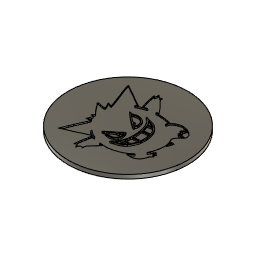
gengar v2 (Autodesk Fusion 360 design; units mm, degrees)
Autodesk Fusion 360 part; units mm, degrees
(part 1 of 2)
sketch "Sketch1" plane through (0, 0, 0) normal (0, 0, 1) x (1, 0, 0)
  circle A0 centre (0, 0) radius 44.85
  dimension "d1" = 89.7
  constraint coincident A0.centre origin
  measures "d1" diameter of A0
extrude "Extrude1" add sketch "Sketch1" along normal blind 2
sketch "Sketch2" plane through (0, 0, 2) normal (0, 0, 1) x (-1, 0, 0)
  circle A0 centre (0, 0) radius 44.85
  line L0 (0, 0) -> (35, 0) construction
  line L1 (35, 0) -> (35, 35) construction
  spline S0 degree 3 poles (24.9655, 28.3529) (24.8458, 28.3933) (24.5786, 28.3486) (24.2945, 28.2347) knots 0 0 0 0 1 1 1 1
  spline S1 degree 3 poles (24.2945, 28.2347) (24.0383, 28.1309) (22.2564, 27.4299) (20.3388, 26.6689) knots 0 0 0 0 1 1 1 1
  spline S2 degree 3 poles (20.3388, 26.6689) (18.4212, 25.908) (16.711, 25.212) (16.545, 25.1201) knots 0 0 0 0 1 1 1 1
  spline S3 degree 3 poles (16.545, 25.1201) (16.3696, 25.0248) (15.5285, 24.6241) (14.6653, 24.2259) knots 0 0 0 0 1 1 1 1
  spline S4 degree 3 poles (14.6653, 24.2259) (11.416, 22.7388) (8.4179, 21.3116) (7.8616, 20.9936) knots 0 0 0 0 1 1 1 1
  line L2 (7.8616, 20.9936) -> (7.5666, 20.8232)
  line L3 (7.5666, 20.8232) -> (7.7132, 21.2861)
  spline S5 degree 3 poles (7.7132, 21.2861) (7.9347, 21.9757) (8.1275, 22.8019) (8.1956, 23.3937) knots 0 0 0 0 1 1 1 1
  spline S6 degree 3 poles (8.1956, 23.3937) (8.2284, 23.6786) (8.3176, 24.0681) (8.3842, 24.2603) knots 0 0 0 0 1 1 1 1
  spline S7 degree 3 poles (8.3842, 24.2603) (8.4507, 24.4526) (8.5341, 24.8294) (8.5702, 25.1051) knots 0 0 0 0 1 1 1 1
  spline S8 degree 3 poles (8.5702, 25.1051) (8.6005, 25.3681) (8.6687, 25.7289) (8.7142, 25.8925) knots 0 0 0 0 1 1 1 1
  spline S9 degree 3 poles (8.7142, 25.8925) (8.8203, 26.2356) (8.9339, 26.991) (8.9994, 27.6763) knots 0 0 0 0 1 1 1 1
  spline S10 degree 3 poles (8.9994, 27.6763) (9.017, 27.9453) (9.0565, 28.3271) (9.0792, 28.5244) knots 0 0 0 0 1 1 1 1
  spline S11 degree 3 poles (9.0792, 28.5244) (9.1078, 28.7343) (9.1111, 28.956) (9.0934, 29.0336) knots 0 0 0 0 1 1 1 1
  spline S12 degree 3 poles (9.0934, 29.0336) (9.0757, 29.1111) (9.0975, 29.3396) (9.1481, 29.547) knots 0 0 0 0 1 1 1 1
  spline S13 degree 3 poles (9.1481, 29.547) (9.1927, 29.7417) (9.2609, 30.1026) (9.2886, 30.3437) knots 0 0 0 0 1 1 1 1
  spline S14 degree 3 poles (9.2886, 30.3437) (9.329, 30.5789) (9.4241, 30.981) (9.4983, 31.239) knots 0 0 0 0 1 1 1 1
  spline S15 degree 3 poles (9.4983, 31.239) (9.6549, 31.7895) (9.5873, 32.3214) (9.3368, 32.5768) knots 0 0 0 0 1 1 1 1
  spline S16 degree 3 poles (9.3368, 32.5768) (9.1024, 32.817) (8.6363, 32.7418) (7.9788, 32.3555) knots 0 0 0 0 1 1 1 1
  spline S17 degree 3 poles (7.9788, 32.3555) (7.7024, 32.1919) (7.4563, 32.0603) (7.4403, 32.0755) knots 0 0 0 0 1 1 1 1
  spline S18 degree 3 poles (7.4403, 32.0755) (7.415, 32.0873) (7.3854, 32.255) (7.3643, 32.4573) knots 0 0 0 0 1 1 1 1
  spline S19 degree 3 poles (7.3643, 32.4573) (7.3507, 32.7254) (7.2647, 32.9041) (7.0547, 33.1637) knots 0 0 0 0 1 1 1 1
  spline S20 degree 3 poles (7.0547, 33.1637) (6.9029, 33.3499) (6.7199, 33.6508) (6.6591, 33.8177) knots 0 0 0 0 1 1 1 1
  line L4 (6.6591, 33.8177) -> (6.5444, 34.133)
  line L5 (6.5444, 34.133) -> (5.7099, 33.8292)
  line L6 (5.7099, 33.8292) -> (4.8847, 33.5289)
  line L7 (4.8847, 33.5289) -> (4.7862, 33.136)
  spline S21 degree 3 poles (4.7862, 33.136) (4.6506, 32.6142) (4.2876, 31.7365) (4.1948, 31.7028) knots 0 0 0 0 1 1 1 1
  spline S22 degree 3 poles (4.1948, 31.7028) (4.1485, 31.6859) (3.807, 31.8451) (3.4268, 32.0532) knots 0 0 0 0 1 1 1 1
  spline S23 degree 3 poles (3.4268, 32.0532) (2.7295, 32.4399) (2.3973, 32.4871) (2.0855, 32.2475) knots 0 0 0 0 1 1 1 1
  spline S24 degree 3 poles (2.0855, 32.2475) (1.9203, 32.1244) (1.8757, 31.8142) (1.754, 30.1003) knots 0 0 0 0 1 1 1 1
  spline S25 degree 3 poles (1.754, 30.1003) (1.7271, 29.7126) (1.6438, 29.4512) (1.4803, 29.2657) knots 0 0 0 0 1 1 1 1
  spline S26 degree 3 poles (1.4803, 29.2657) (1.3437, 29.1215) (1.1424, 28.8382) (1.0387, 28.6325) knots 0 0 0 0 1 1 1 1
  spline S27 degree 3 poles (1.0387, 28.6325) (0.9224, 28.4327) (0.796, 28.2606) (0.7682, 28.2505) knots 0 0 0 0 1 1 1 1
  spline S28 degree 3 poles (0.7682, 28.2505) (0.7311, 28.237) (0.239, 27.7429) (-0.3442, 27.1526) knots 0 0 0 0 1 1 1 1
  spline S29 degree 3 poles (-0.3442, 27.1526) (-0.9181, 26.5657) (-1.4617, 26.0109) (-1.5468, 25.9274) knots 0 0 0 0 1 1 1 1
  spline S30 degree 3 poles (-1.5468, 25.9274) (-1.6319, 25.8439) (-1.792, 25.6491) (-1.9125, 25.4898) knots 0 0 0 0 1 1 1 1
  spline S31 degree 3 poles (-1.9125, 25.4898) (-2.0237, 25.3338) (-2.269, 25.0555) (-2.4451, 24.8759) knots 0 0 0 0 1 1 1 1
  spline S32 degree 3 poles (-2.4451, 24.8759) (-2.6179, 24.687) (-2.7586, 24.4678) (-2.7594, 24.3835) knots 0 0 0 0 1 1 1 1
  spline S33 degree 3 poles (-2.7594, 24.3835) (-2.7602, 24.2992) (-2.8234, 24.2132) (-2.8976, 24.1862) knots 0 0 0 0 1 1 1 1
  spline S34 degree 3 poles (-2.8976, 24.1862) (-2.9718, 24.1592) (-3.212, 23.9248) (-3.4235, 23.6693) knots 0 0 0 0 1 1 1 1
  spline S35 degree 3 poles (-3.4235, 23.6693) (-3.635, 23.4138) (-3.8777, 23.1575) (-3.9822, 23.0984) knots 0 0 0 0 1 1 1 1
  spline S36 degree 3 poles (-3.9822, 23.0984) (-4.0775, 23.0428) (-4.7156, 22.9785) (-5.4018, 22.9598) knots 0 0 0 0 1 1 1 1
  spline S37 degree 3 poles (-5.4018, 22.9598) (-7.9965, 22.8764) (-8.3724, 22.813) (-11.5907, 21.9042) knots 0 0 0 0 1 1 1 1
  spline S38 degree 3 poles (-11.5907, 21.9042) (-13.5606, 21.3447) (-16.0531, 20.3745) (-16.4703, 19.9917) knots 0 0 0 0 1 1 1 1
  spline S39 degree 3 poles (-16.4703, 19.9917) (-16.7964, 19.705) (-17.2542, 19.6644) (-18.0837, 19.8664) knots 0 0 0 0 1 1 1 1
  spline S40 degree 3 poles (-18.0837, 19.8664) (-19.312, 20.1544) (-19.4908, 20.1838) (-20.0969, 20.2047) knots 0 0 0 0 1 1 1 1
  spline S41 degree 3 poles (-20.0969, 20.2047) (-21.2189, 20.2583) (-22.0602, 20.0887) (-23.9517, 19.4002) knots 0 0 0 0 1 1 1 1
  line L8 (-23.9517, 19.4002) -> (-25.7133, 18.759)
  line L9 (-25.7133, 18.759) -> (-26.4592, 18.0675)
  spline S42 degree 3 poles (-26.4592, 18.0675) (-26.8671, 17.6881) (-27.4089, 17.0708) (-27.6643, 16.7049) knots 0 0 0 0 1 1 1 1
  spline S43 degree 3 poles (-27.6643, 16.7049) (-28.1269, 16.043) (-28.896, 14.377) (-28.8285, 14.1916) knots 0 0 0 0 1 1 1 1
  spline S44 degree 3 poles (-28.8285, 14.1916) (-28.8083, 14.136) (-28.8402, 13.8198) (-28.9093, 13.4902) knots 0 0 0 0 1 1 1 1
  spline S45 degree 3 poles (-28.9093, 13.4902) (-28.9968, 13.0383) (-29.1004, 12.8326) (-29.3238, 12.6673) knots 0 0 0 0 1 1 1 1
  spline S46 degree 3 poles (-29.3238, 12.6673) (-29.4797, 12.5476) (-29.7915, 12.1926) (-30.0266, 11.8865) knots 0 0 0 0 1 1 1 1
  spline S47 degree 3 poles (-30.0266, 11.8865) (-30.2491, 11.5745) (-30.4698, 11.3157) (-30.5069, 11.3022) knots 0 0 0 0 1 1 1 1
  spline S48 degree 3 poles (-30.5069, 11.3022) (-30.544, 11.2887) (-30.6923, 11.0037) (-30.8389, 10.6563) knots 0 0 0 0 1 1 1 1
  spline S49 degree 3 poles (-30.8389, 10.6563) (-31.1556, 9.911) (-31.0847, 9.6008) (-30.5764, 9.5023) knots 0 0 0 0 1 1 1 1
  line L10 (-30.5764, 9.5023) -> (-30.2122, 9.4249)
  line L11 (-30.2122, 9.4249) -> (-30.5678, 9.075)
  spline S50 degree 3 poles (-30.5678, 9.075) (-30.8535, 8.7925) (-30.9209, 8.6314) (-30.9435, 8.2032) knots 0 0 0 0 1 1 1 1
  spline S51 degree 3 poles (-30.9435, 8.2032) (-30.9989, 7.259) (-30.8488, 7.1351) (-29.8862, 7.3175) knots 0 0 0 0 1 1 1 1
  spline S52 degree 3 poles (-29.8862, 7.3175) (-29.5414, 7.38) (-29.243, 7.4256) (-29.2303, 7.4197) knots 0 0 0 0 1 1 1 1
  spline S53 degree 3 poles (-29.2303, 7.4197) (-29.205, 7.4079) (-29.2269, 7.1795) (-29.2757, 6.9097) knots 0 0 0 0 1 1 1 1
  spline S54 degree 3 poles (-29.2757, 6.9097) (-29.3153, 6.6433) (-29.3185, 6.3061) (-29.2679, 6.167) knots 0 0 0 0 1 1 1 1
  spline S55 degree 3 poles (-29.2679, 6.167) (-29.089, 5.6756) (-28.3691, 5.7171) (-27.7969, 6.2509) knots 0 0 0 0 1 1 1 1
  spline S56 degree 3 poles (-27.7969, 6.2509) (-27.4649, 6.5503) (-26.965, 6.7637) (-26.911, 6.6153) knots 0 0 0 0 1 1 1 1
  spline S57 degree 3 poles (-26.911, 6.6153) (-26.8908, 6.5597) (-26.9539, 6.3582) (-27.0424, 6.1685) knots 0 0 0 0 1 1 1 1
  spline S58 degree 3 poles (-27.0424, 6.1685) (-27.2513, 5.7039) (-27.6445, 4.1013) (-27.7968, 3.0484) knots 0 0 0 0 1 1 1 1
  spline S59 degree 3 poles (-27.7968, 3.0484) (-27.9752, 1.8074) (-27.9886, 1.6135) (-28.0356, 0.9349) knots 0 0 0 0 1 1 1 1
  spline S60 degree 3 poles (-28.0356, 0.9349) (-28.0734, 0.4906) (-28.1534, 0.22) (-28.338, 0.0058) knots 0 0 0 0 1 1 1 1
  spline S61 degree 3 poles (-28.338, 0.0058) (-28.4736, -0.1696) (-28.5815, -0.3348) (-28.568, -0.3719) knots 0 0 0 0 1 1 1 1
  spline S62 degree 3 poles (-28.568, -0.3719) (-28.5545, -0.409) (-28.632, -0.5422) (-28.7441, -0.667) knots 0 0 0 0 1 1 1 1
  spline S63 degree 3 poles (-28.7441, -0.667) (-28.8562, -0.7918) (-29.0466, -1.1341) (-29.1729, -1.4216) knots 0 0 0 0 1 1 1 1
  spline S64 degree 3 poles (-29.1729, -1.4216) (-29.3052, -1.7218) (-29.5108, -2.1956) (-29.6464, -2.4865) knots 0 0 0 0 1 1 1 1
  spline S65 degree 3 poles (-29.6464, -2.4865) (-30.3406, -4.0411) (-30.3889, -5.9278) (-29.7296, -6.1813) knots 0 0 0 0 1 1 1 1
  spline S66 degree 3 poles (-29.7296, -6.1813) (-29.6158, -6.2344) (-29.0653, -6.2755) (-28.5123, -6.2948) knots 0 0 0 0 1 1 1 1
  spline S67 degree 3 poles (-28.5123, -6.2948) (-26.6256, -6.3431) (-26.4461, -6.4037) (-26.0437, -7.1918) knots 0 0 0 0 1 1 1 1
  spline S68 degree 3 poles (-26.0437, -7.1918) (-25.8194, -7.6352) (-25.8126, -7.6537) (-26.0511, -8.066) knots 0 0 0 0 1 1 1 1
  spline S69 degree 3 poles (-26.0511, -8.066) (-26.1884, -8.2945) (-26.3754, -8.6461) (-26.4791, -8.8518) knots 0 0 0 0 1 1 1 1
  spline S70 degree 3 poles (-26.4791, -8.8518) (-26.6383, -9.1933) (-28.4257, -11.0619) (-29.2104, -11.7045) knots 0 0 0 0 1 1 1 1
  spline S71 degree 3 poles (-29.2104, -11.7045) (-30.065, -12.4145) (-30.5646, -13.3209) (-30.5585, -14.1167) knots 0 0 0 0 1 1 1 1
  spline S72 degree 3 poles (-30.5585, -14.1167) (-30.555, -14.3569) (-30.3381, -15.097) (-29.9661, -16.1481) knots 0 0 0 0 1 1 1 1
  spline S73 degree 3 poles (-29.9661, -16.1481) (-29.3814, -17.7834) (-29.3654, -17.7985) (-28.9564, -18.1432) knots 0 0 0 0 1 1 1 1
  spline S74 degree 3 poles (-28.9564, -18.1432) (-28.7296, -18.3336) (-28.4842, -18.5173) (-28.4083, -18.5527) knots 0 0 0 0 1 1 1 1
  spline S75 degree 3 poles (-28.4083, -18.5527) (-28.3417, -18.5915) (-28.0205, -18.8106) (-27.7085, -19.033) knots 0 0 0 0 1 1 1 1
  spline S76 degree 3 poles (-27.7085, -19.033) (-26.5146, -19.89) (-23.9634, -20.841) (-22.4266, -20.9956) knots 0 0 0 0 1 1 1 1
  spline S77 degree 3 poles (-22.4266, -20.9956) (-21.9789, -21.0427) (-21.522, -21.0864) (-21.4251, -21.0931) knots 0 0 0 0 1 1 1 1
  spline S78 degree 3 poles (-21.4251, -21.0931) (-20.7169, -21.1924) (-18.0254, -20.6538) (-17.2028, -20.2599) knots 0 0 0 0 1 1 1 1
  spline S79 degree 3 poles (-17.2028, -20.2599) (-15.8904, -19.6247) (-15.1007, -19.1692) (-14.6835, -18.7864) knots 0 0 0 0 1 1 1 1
  spline S80 degree 3 poles (-14.6835, -18.7864) (-14.0986, -18.2585) (-14.0708, -18.2484) (-13.6973, -18.438) knots 0 0 0 0 1 1 1 1
  spline S81 degree 3 poles (-13.6973, -18.438) (-13.5295, -18.5239) (-13.344, -18.5719) (-13.2791, -18.5483) knots 0 0 0 0 1 1 1 1
  spline S82 degree 3 poles (-13.2791, -18.5483) (-13.2142, -18.5246) (-13.0827, -18.5398) (-12.9815, -18.587) knots 0 0 0 0 1 1 1 1
  spline S83 degree 3 poles (-12.9815, -18.587) (-12.447, -18.8439) (-6.9732, -19.7182) (-6.6672, -19.6068) knots 0 0 0 0 1 1 1 1
  spline S84 degree 3 poles (-6.6672, -19.6068) (-6.6116, -19.5866) (-6.2769, -19.6117) (-5.9355, -19.6555) knots 0 0 0 0 1 1 1 1
  spline S85 degree 3 poles (-5.9355, -19.6555) (-5.5907, -19.7085) (-5.2686, -19.7278) (-5.2037, -19.7042) knots 0 0 0 0 1 1 1 1
  spline S86 degree 3 poles (-5.2037, -19.7042) (-4.9905, -19.6265) (-4.6869, -19.8836) (-4.159, -20.5839) knots 0 0 0 0 1 1 1 1
  spline S87 degree 3 poles (-4.159, -20.5839) (-3.0509, -22.0707) (-2.4665, -22.782) (-2.0659, -23.1612) knots 0 0 0 0 1 1 1 1
  spline S88 degree 3 poles (-2.0659, -23.1612) (-1.8416, -23.3736) (-1.619, -23.639) (-1.5819, -23.741) knots 0 0 0 0 1 1 1 1
  spline S89 degree 3 poles (-1.5819, -23.741) (-1.5448, -23.843) (-1.1552, -24.2787) (-0.7125, -24.7161) knots 0 0 0 0 1 1 1 1
  spline S90 degree 3 poles (-0.7125, -24.7161) (-0.2731, -25.1442) (0.151, -25.5884) (0.2354, -25.7047) knots 0 0 0 0 1 1 1 1
  spline S91 degree 3 poles (0.2354, -25.7047) (0.3197, -25.821) (0.5474, -26.0426) (0.7329, -26.2061) knots 0 0 0 0 1 1 1 1
  spline S92 degree 3 poles (0.7329, -26.2061) (0.9276, -26.3662) (1.227, -26.6983) (1.4142, -26.9241) knots 0 0 0 0 1 1 1 1
  spline S93 degree 3 poles (1.4142, -26.9241) (1.5955, -27.1627) (1.7853, -27.3666) (1.8418, -27.3776) knots 0 0 0 0 1 1 1 1
  spline S94 degree 3 poles (1.8418, -27.3776) (2.0238, -27.4163) (3.6066, -29.0242) (3.6235, -29.1861) knots 0 0 0 0 1 1 1 1
  spline S95 degree 3 poles (3.6235, -29.1861) (3.6261, -29.2797) (3.6372, -29.6851) (3.6356, -30.0847) knots 0 0 0 0 1 1 1 1
  spline S96 degree 3 poles (3.6356, -30.0847) (3.635, -30.862) (3.7927, -31.2666) (4.0962, -31.2926) knots 0 0 0 0 1 1 1 1
  spline S97 degree 3 poles (4.0962, -31.2926) (4.1966, -31.3086) (4.6989, -31.1887) (5.219, -31.0309) knots 0 0 0 0 1 1 1 1
  line L12 (5.219, -31.0309) -> (6.1631, -30.7398)
  line L13 (6.1631, -30.7398) -> (6.648, -31.3509)
  spline S98 degree 3 poles (6.648, -31.3509) (7.482, -32.4018) (8.1363, -32.8147) (8.5029, -32.5238) knots 0 0 0 0 1 1 1 1
  spline S99 degree 3 poles (8.5029, -32.5238) (8.6833, -32.3846) (8.9839, -31.1622) (8.9812, -30.6066) knots 0 0 0 0 1 1 1 1
  spline S100 degree 3 poles (8.9812, -30.6066) (8.982, -30.4069) (8.9785, -30.1666) (8.9793, -30.0823) knots 0 0 0 0 1 1 1 1
  spline S101 degree 3 poles (8.9793, -30.0823) (8.9827, -29.9761) (9.1092, -30.0351) (9.3655, -30.2778) knots 0 0 0 0 1 1 1 1
  spline S102 degree 3 poles (9.3655, -30.2778) (9.6859, -30.5811) (9.7964, -30.625) (10.0189, -30.544) knots 0 0 0 0 1 1 1 1
  spline S103 degree 3 poles (10.0189, -30.544) (10.4639, -30.382) (10.5161, -30.006) (10.3385, -28.1911) knots 0 0 0 0 1 1 1 1
  spline S104 degree 3 poles (10.3385, -28.1911) (10.2794, -27.6246) (9.8396, -25.6951) (9.6405, -25.1481) knots 0 0 0 0 1 1 1 1
  spline S105 degree 3 poles (9.6405, -25.1481) (9.546, -24.8884) (9.5012, -24.6212) (9.5375, -24.5765) knots 0 0 0 0 1 1 1 1
  spline S106 degree 3 poles (9.5375, -24.5765) (9.583, -24.5285) (9.4615, -24.0792) (9.2725, -23.56) knots 0 0 0 0 1 1 1 1
  spline S107 degree 3 poles (9.2725, -23.56) (9.0869, -23.05) (8.8885, -22.3032) (8.8243, -21.896) knots 0 0 0 0 1 1 1 1
  spline S108 degree 3 poles (8.8243, -21.896) (8.7694, -21.4855) (8.5576, -20.5861) (8.3576, -19.8924) knots 0 0 0 0 1 1 1 1
  spline S109 degree 3 poles (8.3576, -19.8924) (7.95, -18.4552) (7.7837, -17.6232) (7.878, -17.4208) knots 0 0 0 0 1 1 1 1
  spline S110 degree 3 poles (7.878, -17.4208) (7.9522, -17.2784) (8.5086, -17.5378) (10.0212, -18.4048) knots 0 0 0 0 1 1 1 1
  spline S111 degree 3 poles (10.0212, -18.4048) (10.4209, -18.6374) (11.0895, -19.003) (11.5009, -19.2103) knots 0 0 0 0 1 1 1 1
  spline S112 degree 3 poles (11.5009, -19.2103) (11.9031, -19.4209) (12.2488, -19.6206) (12.2589, -19.6484) knots 0 0 0 0 1 1 1 1
  spline S113 degree 3 poles (12.2589, -19.6484) (12.2724, -19.6855) (12.4629, -19.8052) (12.6754, -19.9273) knots 0 0 0 0 1 1 1 1
  spline S114 degree 3 poles (12.6754, -19.9273) (12.8972, -20.0461) (13.2521, -20.2424) (13.4646, -20.3646) knots 0 0 0 0 1 1 1 1
  spline S115 degree 3 poles (13.4646, -20.3646) (13.6863, -20.4834) (14.2538, -20.8019) (14.7259, -21.0606) knots 0 0 0 0 1 1 1 1
  spline S116 degree 3 poles (14.7259, -21.0606) (15.2073, -21.3158) (15.7276, -21.62) (15.8996, -21.7464) knots 0 0 0 0 1 1 1 1
  spline S117 degree 3 poles (15.8996, -21.7464) (16.2149, -21.9781) (18.6921, -23.4181) (19.3438, -23.7374) knots 0 0 0 0 1 1 1 1
  spline S118 degree 3 poles (19.3438, -23.7374) (19.5402, -23.8444) (19.8724, -24.007) (20.0655, -24.1047) knots 0 0 0 0 1 1 1 1
  spline S119 degree 3 poles (20.0655, -24.1047) (20.2712, -24.2084) (21.0983, -24.6633) (21.9128, -25.1124) knots 0 0 0 0 1 1 1 1
  spline S120 degree 3 poles (21.9128, -25.1124) (22.7214, -25.5741) (23.6117, -26.0586) (23.884, -26.201) knots 0 0 0 0 1 1 1 1
  spline S121 degree 3 poles (23.884, -26.201) (24.1564, -26.3434) (24.572, -26.5911) (24.8014, -26.7596) knots 0 0 0 0 1 1 1 1
  spline S122 degree 3 poles (24.8014, -26.7596) (25.0307, -26.9281) (25.3258, -27.1042) (25.4582, -27.1506) knots 0 0 0 0 1 1 1 1
  spline S123 degree 3 poles (25.4582, -27.1506) (25.8654, -27.3174) (26.748, -27.4056) (26.8947, -27.2892) knots 0 0 0 0 1 1 1 1
  spline S124 degree 3 poles (26.8947, -27.2892) (26.968, -27.231) (27.0708, -26.9941) (27.1331, -26.7615) knots 0 0 0 0 1 1 1 1
  line L14 (27.1331, -26.7615) -> (27.24, -26.334)
  line L15 (27.24, -26.334) -> (24.1092, -17.7608)
  spline S125 degree 3 poles (24.1092, -17.7608) (21.5157, -10.6931) (20.8965, -9.0494) (20.5329, -8.4257) knots 0 0 0 0 1 1 1 1
  spline S126 degree 3 poles (20.5329, -8.4257) (20.1163, -7.6849) (20.0808, -7.4143) (20.4434, -7.7758) knots 0 0 0 0 1 1 1 1
  spline S127 degree 3 poles (20.4434, -7.7758) (20.5395, -7.8668) (20.7958, -7.994) (21.01, -8.0631) knots 0 0 0 0 1 1 1 1
  spline S128 degree 3 poles (21.01, -8.0631) (21.2241, -8.1322) (21.7308, -8.2838) (22.1372, -8.4194) knots 0 0 0 0 1 1 1 1
  spline S129 degree 3 poles (22.1372, -8.4194) (22.9178, -8.6602) (23.3317, -8.6146) (23.4564, -8.2647) knots 0 0 0 0 1 1 1 1
  spline S130 degree 3 poles (23.4564, -8.2647) (23.5145, -8.107) (23.4276, -7.8972) (22.957, -7.0079) knots 0 0 0 0 1 1 1 1
  spline S131 degree 3 poles (22.957, -7.0079) (22.6382, -6.4205) (22.3134, -5.7302) (22.2189, -5.4705) knots 0 0 0 0 1 1 1 1
  spline S132 degree 3 poles (22.2189, -5.4705) (22.1278, -5.2202) (21.8486, -4.7128) (21.6108, -4.3478) knots 0 0 0 0 1 1 1 1
  line L16 (21.6108, -4.3478) -> (21.1807, -3.6854)
  line L17 (21.1807, -3.6854) -> (21.4294, -3.7629)
  spline S133 degree 3 poles (21.4294, -3.7629) (21.5617, -3.8092) (21.8846, -3.8597) (22.135, -3.884) knots 0 0 0 0 1 1 1 1
  spline S134 degree 3 poles (22.135, -3.884) (22.3854, -3.9084) (22.6298, -3.9454) (22.6653, -3.985) knots 0 0 0 0 1 1 1 1
  spline S135 degree 3 poles (22.6653, -3.985) (22.796, -4.0845) (24.2982, -4.3462) (25.7482, -4.522) knots 0 0 0 0 1 1 1 1
  spline S136 degree 3 poles (25.7482, -4.522) (27.5051, -4.733) (27.8642, -4.6233) (27.676, -3.9043) knots 0 0 0 0 1 1 1 1
  spline S137 degree 3 poles (27.676, -3.9043) (27.6203, -3.6936) (27.3968, -3.2814) (27.1826, -2.9814) knots 0 0 0 0 1 1 1 1
  spline S138 degree 3 poles (27.1826, -2.9814) (26.9591, -2.6847) (26.5079, -2.0509) (26.1638, -1.5671) knots 0 0 0 0 1 1 1 1
  spline S139 degree 3 poles (26.1638, -1.5671) (25.0346, 0.0064) (22.7796, 2.7977) (22.0519, 3.4989) knots 0 0 0 0 1 1 1 1
  spline S140 degree 3 poles (22.0519, 3.4989) (21.0645, 4.452) (20.6268, 4.9332) (20.6521, 5.0369) knots 0 0 0 0 1 1 1 1
  spline S141 degree 3 poles (20.6521, 5.0369) (20.663, 5.0934) (20.8593, 5.3329) (21.0995, 5.5673) knots 0 0 0 0 1 1 1 1
  spline S142 degree 3 poles (21.0995, 5.5673) (21.3304, 5.7984) (21.6346, 6.2031) (21.7711, 6.4628) knots 0 0 0 0 1 1 1 1
  spline S143 degree 3 poles (21.7711, 6.4628) (22.1865, 7.2545) (21.8998, 7.5806) (20.5906, 7.7446) knots 0 0 0 0 1 1 1 1
  spline S144 degree 3 poles (20.5906, 7.7446) (20.3275, 7.7749) (20.1109, 7.822) (20.1007, 7.8498) knots 0 0 0 0 1 1 1 1
  spline S145 degree 3 poles (20.1007, 7.8498) (20.094, 7.8684) (20.1757, 8.0766) (20.2819, 8.3043) knots 0 0 0 0 1 1 1 1
  spline S146 degree 3 poles (20.2819, 8.3043) (20.3787, 8.5285) (20.623, 9.069) (20.8168, 9.5175) knots 0 0 0 0 1 1 1 1
  spline S147 degree 3 poles (20.8168, 9.5175) (21.0047, 9.9534) (21.2877, 10.5604) (21.4512, 10.8614) knots 0 0 0 0 1 1 1 1
  spline S148 degree 3 poles (21.4512, 10.8614) (21.6054, 11.159) (21.7115, 11.5022) (21.6862, 11.6295) knots 0 0 0 0 1 1 1 1
  spline S149 degree 3 poles (21.6862, 11.6295) (21.5899, 12.0669) (21.305, 12.0997) (20.0178, 11.7993) knots 0 0 0 0 1 1 1 1
  spline S150 degree 3 poles (20.0178, 11.7993) (18.5663, 11.4599) (18.4449, 11.4473) (18.6691, 11.6969) knots 0 0 0 0 1 1 1 1
  spline S151 degree 3 poles (18.6691, 11.6969) (18.7567, 11.8023) (18.9547, 12.2103) (19.1248, 12.6083) knots 0 0 0 0 1 1 1 1
  spline S152 degree 3 poles (19.1248, 12.6083) (19.2824, 13.0121) (19.4854, 13.464) (19.5688, 13.6099) knots 0 0 0 0 1 1 1 1
  spline S153 degree 3 poles (19.5688, 13.6099) (19.6581, 13.7684) (19.771, 13.9775) (19.8114, 14.0972) knots 0 0 0 0 1 1 1 1
  spline S154 degree 3 poles (19.8114, 14.0972) (19.8645, 14.211) (20.1644, 14.8872) (20.482, 15.6013) knots 0 0 0 0 1 1 1 1
  spline S155 degree 3 poles (20.482, 15.6013) (21.1762, 17.156) (22.182, 19.5276) (23.1019, 21.7315) knots 0 0 0 0 1 1 1 1
  spline S156 degree 3 poles (23.1019, 21.7315) (23.465, 22.6091) (23.8576, 23.55) (23.9662, 23.7996) knots 0 0 0 0 1 1 1 1
  spline S157 degree 3 poles (23.9662, 23.7996) (24.3032, 24.6048) (24.5786, 25.377) (24.7176, 25.8896) knots 0 0 0 0 1 1 1 1
  spline S158 degree 3 poles (24.7176, 25.8896) (24.7976, 26.1602) (24.9508, 26.72) (25.0864, 27.1264) knots 0 0 0 0 1 1 1 1
  spline S159 degree 3 poles (25.0864, 27.1264) (25.3214, 27.8944) (25.2935, 28.2308) (24.9655, 28.3529) knots 0 0 0 0 1 1 1 1
  spline S160 degree 3 poles (24.385, 27.2071) (24.3243, 27.2585) (24.2586, 27.2661) (24.2468, 27.2408) knots 0 0 0 0 1 1 1 1
  spline S161 degree 3 poles (24.2468, 27.2408) (24.2384, 27.2062) (24.0674, 26.724) (23.8737, 26.16) knots 0 0 0 0 1 1 1 1
  spline S162 degree 3 poles (23.8737, 26.16) (23.5527, 25.2241) (22.4636, 22.4757) (22.3001, 22.1747) knots 0 0 0 0 1 1 1 1
  spline S163 degree 3 poles (22.3001, 22.1747) (22.2555, 22.0954) (21.7896, 20.9808) (21.2505, 19.6926) knots 0 0 0 0 1 1 1 1
  spline S164 degree 3 poles (21.2505, 19.6926) (20.2725, 17.3311) (19.5412, 15.6474) (18.8748, 14.2183) knots 0 0 0 0 1 1 1 1
  spline S165 degree 3 poles (18.8748, 14.2183) (18.6743, 13.7883) (18.3424, 13.027) (18.1377, 12.522) knots 0 0 0 0 1 1 1 1
  spline S166 degree 3 poles (18.1377, 12.522) (17.933, 12.017) (17.6963, 11.4268) (17.6146, 11.2186) knots 0 0 0 0 1 1 1 1
  spline S167 degree 3 poles (17.6146, 11.2186) (17.3695, 10.5938) (17.3662, 10.3721) (17.6268, 9.858) knots 0 0 0 0 1 1 1 1
  spline S168 degree 3 poles (17.6268, 9.858) (17.96, 9.2022) (18.1818, 8.9679) (18.4043, 9.0489) knots 0 0 0 0 1 1 1 1
  spline S169 degree 3 poles (18.4043, 9.0489) (18.6361, 9.1333) (18.6073, 9.5008) (18.318, 10.036) knots 0 0 0 0 1 1 1 1
  line L18 (18.318, 10.036) -> (18.1071, 10.4423)
  line L19 (18.1071, 10.4423) -> (19.0731, 10.7309)
  spline S170 degree 3 poles (19.0731, 10.7309) (20.0762, 11.033) (20.4243, 11.0862) (20.4286, 10.9302) knots 0 0 0 0 1 1 1 1
  spline S171 degree 3 poles (20.4286, 10.9302) (20.4236, 10.8864) (20.1894, 10.3182) (19.8979, 9.6766) knots 0 0 0 0 1 1 1 1
  spline S172 degree 3 poles (19.8979, 9.6766) (19.074, 7.8436) (18.829, 6.7569) (19.2555, 6.7967) knots 0 0 0 0 1 1 1 1
  spline S173 degree 3 poles (19.2555, 6.7967) (19.8127, 6.8525) (20.8867, 6.8444) (20.907, 6.7888) knots 0 0 0 0 1 1 1 1
  spline S174 degree 3 poles (20.907, 6.7888) (20.9205, 6.7517) (20.6516, 6.4228) (20.312, 6.0577) knots 0 0 0 0 1 1 1 1
  spline S175 degree 3 poles (20.312, 6.0577) (19.5047, 5.2178) (19.4718, 5.1639) (19.6523, 4.8411) knots 0 0 0 0 1 1 1 1
  spline S176 degree 3 poles (19.6523, 4.8411) (19.8067, 4.5612) (20.9114, 3.3148) (21.4974, 2.7721) knots 0 0 0 0 1 1 1 1
  spline S177 degree 3 poles (21.4974, 2.7721) (22.0421, 2.2563) (24.5223, -0.8941) (26.08, -3.0677) knots 0 0 0 0 1 1 1 1
  spline S178 degree 3 poles (26.08, -3.0677) (26.5666, -3.7411) (26.5868, -3.7967) (26.328, -3.6914) knots 0 0 0 0 1 1 1 1
  spline S179 degree 3 poles (26.328, -3.6914) (26.2049, -3.6417) (26.0042, -3.6098) (25.8829, -3.6225) knots 0 0 0 0 1 1 1 1
  spline S180 degree 3 poles (25.8829, -3.6225) (25.6645, -3.6284) (23.2526, -3.2043) (22.031, -2.9349) knots 0 0 0 0 1 1 1 1
  spline S181 degree 3 poles (22.031, -2.9349) (21.29, -2.7741) (20.2025, -2.7289) (20.1402, -2.8461) knots 0 0 0 0 1 1 1 1
  spline S182 degree 3 poles (20.1402, -2.8461) (20.0635, -3.0105) (20.4094, -4.0186) (20.794, -4.7291) knots 0 0 0 0 1 1 1 1
  spline S183 degree 3 poles (20.794, -4.7291) (20.9981, -5.1168) (21.3246, -5.754) (21.5194, -6.1451) knots 0 0 0 0 1 1 1 1
  spline S184 degree 3 poles (21.5194, -6.1451) (21.7143, -6.5362) (21.9614, -7.0133) (22.0635, -7.2072) knots 0 0 0 0 1 1 1 1
  line L20 (22.0635, -7.2072) -> (22.2541, -7.5578)
  line L21 (22.2541, -7.5578) -> (21.9531, -7.3943)
  spline S185 degree 3 poles (21.9531, -7.3943) (21.6394, -7.225) (20.3613, -6.8291) (20.2501, -6.8696) knots 0 0 0 0 1 1 1 1
  spline S186 degree 3 poles (20.2501, -6.8696) (20.111, -6.9203) (19.7274, -6.7029) (19.6666, -6.536) knots 0 0 0 0 1 1 1 1
  spline S187 degree 3 poles (19.6666, -6.536) (19.5823, -6.3042) (19.2923, -6.3152) (19.1769, -6.5463) knots 0 0 0 0 1 1 1 1
  spline S188 degree 3 poles (19.1769, -6.5463) (19.1002, -6.7107) (19.3145, -7.3572) (20.769, -11.3534) knots 0 0 0 0 1 1 1 1
  spline S189 degree 3 poles (20.769, -11.3534) (21.6903, -13.8846) (22.9102, -17.0632) (23.4746, -18.4118) knots 0 0 0 0 1 1 1 1
  spline S190 degree 3 poles (23.4746, -18.4118) (24.033, -19.7731) (24.7695, -21.7101) (25.1062, -22.7216) knots 0 0 0 0 1 1 1 1
  spline S191 degree 3 poles (25.1062, -22.7216) (25.7145, -24.5372) (26.1728, -26.3445) (26.0337, -26.3951) knots 0 0 0 0 1 1 1 1
  spline S192 degree 3 poles (26.0337, -26.3951) (25.9966, -26.4086) (25.8542, -26.3344) (25.7108, -26.2291) knots 0 0 0 0 1 1 1 1
  spline S193 degree 3 poles (25.7108, -26.2291) (25.5734, -26.1111) (25.269, -25.9384) (25.0414, -25.8322) knots 0 0 0 0 1 1 1 1
  spline S194 degree 3 poles (25.0414, -25.8322) (24.8137, -25.7261) (24.275, -25.4287) (23.8525, -25.1624) knots 0 0 0 0 1 1 1 1
  spline S195 degree 3 poles (23.8525, -25.1624) (22.8559, -24.5591) (20.2701, -23.1378) (18.9531, -22.4621) knots 0 0 0 0 1 1 1 1
  spline S196 degree 3 poles (18.9531, -22.4621) (18.3865, -22.1748) (17.4827, -21.6532) (16.9363, -21.3061) knots 0 0 0 0 1 1 1 1
  spline S197 degree 3 poles (16.9363, -21.3061) (16.3992, -20.9555) (15.3267, -20.3169) (14.5629, -19.8914) knots 0 0 0 0 1 1 1 1
  spline S198 degree 3 poles (14.5629, -19.8914) (13.7956, -19.4566) (12.7746, -18.8727) (12.2889, -18.577) knots 0 0 0 0 1 1 1 1
  spline S199 degree 3 poles (12.2889, -18.577) (11.8066, -18.2905) (11.0934, -17.8886) (10.7106, -17.7024) knots 0 0 0 0 1 1 1 1
  spline S200 degree 3 poles (10.7106, -17.7024) (9.5429, -17.1194) (9.0075, -16.8313) (9.0252, -16.7933) knots 0 0 0 0 1 1 1 1
  spline S201 degree 3 poles (9.0252, -16.7933) (9.037, -16.768) (9.3008, -16.5985) (9.605, -16.4248) knots 0 0 0 0 1 1 1 1
  spline S202 degree 3 poles (9.605, -16.4248) (10.4588, -15.9145) (10.5616, -15.7931) (10.4166, -15.5099) knots 0 0 0 0 1 1 1 1
  spline S203 degree 3 poles (10.4166, -15.5099) (10.3078, -15.2975) (10.2605, -15.2832) (9.9765, -15.397) knots 0 0 0 0 1 1 1 1
  spline S204 degree 3 poles (9.9765, -15.397) (9.8003, -15.4612) (9.3486, -15.7201) (8.9743, -15.9613) knots 0 0 0 0 1 1 1 1
  spline S205 degree 3 poles (8.9743, -15.9613) (8.3085, -16.3821) (7.3822, -16.7508) (3.9119, -17.9194) knots 0 0 0 0 1 1 1 1
  spline S206 degree 3 poles (3.9119, -17.9194) (3.4078, -18.0923) (3.3589, -18.1311) (3.3952, -18.3174) knots 0 0 0 0 1 1 1 1
  spline S207 degree 3 poles (3.3952, -18.3174) (3.4628, -18.6184) (3.6524, -18.5913) (5.2683, -18.0977) knots 0 0 0 0 1 1 1 1
  spline S208 degree 3 poles (5.2683, -18.0977) (6.0607, -17.8513) (6.7392, -17.6673) (6.7898, -17.6909) knots 0 0 0 0 1 1 1 1
  spline S209 degree 3 poles (6.7898, -17.6909) (6.837, -17.7052) (7.0286, -18.318) (7.2294, -19.043) knots 0 0 0 0 1 1 1 1
  spline S210 degree 3 poles (7.2294, -19.043) (7.4269, -19.7586) (7.8682, -21.404) (8.2218, -22.6928) knots 0 0 0 0 1 1 1 1
  spline S211 degree 3 poles (8.2218, -22.6928) (8.5754, -23.9817) (8.9527, -25.4509) (9.054, -25.96) knots 0 0 0 0 1 1 1 1
  spline S212 degree 3 poles (9.054, -25.96) (9.5538, -28.4872) (9.6323, -28.9626) (9.6096, -29.1599) knots 0 0 0 0 1 1 1 1
  spline S213 degree 3 poles (9.6096, -29.1599) (9.5836, -29.3479) (9.565, -29.3546) (9.3787, -29.2754) knots 0 0 0 0 1 1 1 1
  spline S214 degree 3 poles (9.3787, -29.2754) (9.2109, -29.1895) (9.178, -29.128) (9.1712, -28.763) knots 0 0 0 0 1 1 1 1
  spline S215 degree 3 poles (9.1712, -28.763) (9.1618, -28.5354) (9.1053, -28.2934) (9.0505, -28.2294) knots 0 0 0 0 1 1 1 1
  spline S216 degree 3 poles (9.0505, -28.2294) (8.9214, -28.0768) (8.6492, -28.1654) (8.5118, -28.3939) knots 0 0 0 0 1 1 1 1
  spline S217 degree 3 poles (8.5118, -28.3939) (8.3593, -28.6384) (8.0908, -30.1222) (8.1685, -30.3354) knots 0 0 0 0 1 1 1 1
  spline S218 degree 3 poles (8.1685, -30.3354) (8.1929, -30.4315) (8.1888, -30.7375) (8.1526, -31.0132) knots 0 0 0 0 1 1 1 1
  line L22 (8.1526, -31.0132) -> (8.0912, -31.5081)
  line L23 (8.0912, -31.5081) -> (7.7986, -31.1946)
  spline S219 degree 3 poles (7.7986, -31.1946) (6.425, -29.6995) (6.3617, -29.67) (5.2769, -30.0648) knots 0 0 0 0 1 1 1 1
  line L24 (5.2769, -30.0648) -> (4.5073, -30.3449)
  line L25 (4.5073, -30.3449) -> (4.5392, -29.6823)
  spline S220 degree 3 poles (4.5392, -29.6823) (4.5676, -28.895) (4.4048, -28.5342) (3.7058, -27.8541) knots 0 0 0 0 1 1 1 1
  spline S221 degree 3 poles (3.7058, -27.8541) (3.446, -27.6022) (2.8718, -27.0341) (2.435, -26.5841) knots 0 0 0 0 1 1 1 1
  spline S222 degree 3 poles (2.435, -26.5841) (1.9982, -26.1341) (1.2081, -25.3191) (0.6591, -24.7629) knots 0 0 0 0 1 1 1 1
  spline S223 degree 3 poles (0.6591, -24.7629) (0.1135, -24.216) (-0.6361, -23.3968) (-1.0165, -22.9577) knots 0 0 0 0 1 1 1 1
  spline S224 degree 3 poles (-1.0165, -22.9577) (-1.8319, -22.0155) (-3.7462, -19.5832) (-3.7167, -19.5199) knots 0 0 0 0 1 1 1 1
  spline S225 degree 3 poles (-3.7167, -19.5199) (-3.7142, -19.498) (-3.4285, -19.4465) (-3.1048, -19.4127) knots 0 0 0 0 1 1 1 1
  spline S226 degree 3 poles (-3.1048, -19.4127) (-2.7718, -19.3755) (-2.3807, -19.2962) (-2.2382, -19.2548) knots 0 0 0 0 1 1 1 1
  spline S227 degree 3 poles (-2.2382, -19.2548) (-1.9508, -19.1502) (-1.8986, -18.8897) (-2.1364, -18.7557) knots 0 0 0 0 1 1 1 1
  spline S228 degree 3 poles (-2.1364, -18.7557) (-2.289, -18.6538) (-3.2626, -18.6616) (-3.9184, -18.7638) knots 0 0 0 0 1 1 1 1
  spline S229 degree 3 poles (-3.9184, -18.7638) (-4.1081, -18.7909) (-4.6797, -18.7784) (-5.1897, -18.733) knots 0 0 0 0 1 1 1 1
  spline S230 degree 3 poles (-5.1897, -18.733) (-6.1878, -18.6448) (-6.2502, -18.6465) (-7.1219, -18.6173) knots 0 0 0 0 1 1 1 1
  spline S231 degree 3 poles (-7.1219, -18.6173) (-7.8249, -18.5897) (-9.4039, -18.3768) (-10.0607, -18.2169) knots 0 0 0 0 1 1 1 1
  spline S232 degree 3 poles (-10.0607, -18.2169) (-10.3245, -18.1554) (-10.9771, -18.0359) (-11.5225, -17.9509) knots 0 0 0 0 1 1 1 1
  spline S233 degree 3 poles (-11.5225, -17.9509) (-12.4532, -17.8171) (-13.6031, -17.5427) (-13.6335, -17.4592) knots 0 0 0 0 1 1 1 1
  spline S234 degree 3 poles (-13.6335, -17.4592) (-13.6403, -17.4407) (-13.5518, -17.1355) (-13.4272, -16.7856) knots 0 0 0 0 1 1 1 1
  spline S235 degree 3 poles (-13.4272, -16.7856) (-13.1408, -15.9569) (-13.0947, -15.0161) (-13.3317, -14.7978) knots 0 0 0 0 1 1 1 1
  spline S236 degree 3 poles (-13.3317, -14.7978) (-13.5332, -14.6191) (-13.7447, -14.7591) (-13.7269, -15.0677) knots 0 0 0 0 1 1 1 1
  spline S237 degree 3 poles (-13.7269, -15.0677) (-13.7041, -15.4479) (-14.2052, -16.9848) (-14.4327, -17.2251) knots 0 0 0 0 1 1 1 1
  spline S238 degree 3 poles (-14.4327, -17.2251) (-14.5448, -17.3499) (-15.0387, -17.7817) (-15.5241, -18.1789) knots 0 0 0 0 1 1 1 1
  line L26 (-15.5241, -18.1789) -> (-16.4158, -18.9024)
  line L27 (-16.4158, -18.9024) -> (-18.1775, -19.5436)
  spline S239 degree 3 poles (-18.1775, -19.5436) (-19.661, -20.0836) (-20.0327, -20.1874) (-20.5132, -20.1942) knots 0 0 0 0 1 1 1 1
  spline S240 degree 3 poles (-20.5132, -20.1942) (-21.2028, -20.2037) (-22.8011, -20.082) (-23.0187, -20.0036) knots 0 0 0 0 1 1 1 1
  spline S241 degree 3 poles (-23.0187, -20.0036) (-23.2143, -19.9278) (-24.0135, -19.6937) (-24.7115, -19.5067) knots 0 0 0 0 1 1 1 1
  spline S242 degree 3 poles (-24.7115, -19.5067) (-25.391, -19.3131) (-26.4238, -18.87) (-26.6481, -18.6576) knots 0 0 0 0 1 1 1 1
  spline S243 degree 3 poles (-26.6481, -18.6576) (-26.7535, -18.5699) (-27.0335, -18.3778) (-27.2746, -18.2346) knots 0 0 0 0 1 1 1 1
  spline S244 degree 3 poles (-27.2746, -18.2346) (-27.9601, -17.8226) (-28.7536, -17.1138) (-29.053, -16.6663) knots 0 0 0 0 1 1 1 1
  spline S245 degree 3 poles (-29.053, -16.6663) (-29.1997, -16.4362) (-29.4384, -15.9246) (-29.5743, -15.5225) knots 0 0 0 0 1 1 1 1
  spline S246 degree 3 poles (-29.5743, -15.5225) (-29.8139, -14.8642) (-29.824, -14.7209) (-29.729, -14.0878) knots 0 0 0 0 1 1 1 1
  spline S247 degree 3 poles (-29.729, -14.0878) (-29.6153, -13.4479) (-29.5682, -13.3467) (-29.0583, -12.8147) knots 0 0 0 0 1 1 1 1
  spline S248 degree 3 poles (-29.0583, -12.8147) (-28.7515, -12.5035) (-28.3133, -12.092) (-28.0967, -11.9081) knots 0 0 0 0 1 1 1 1
  spline S249 degree 3 poles (-28.0967, -11.9081) (-27.4621, -11.3727) (-25.9865, -9.7436) (-25.6638, -9.2166) knots 0 0 0 0 1 1 1 1
  spline S250 degree 3 poles (-25.6638, -9.2166) (-25.4961, -8.9561) (-25.2712, -8.5067) (-25.1414, -8.2284) knots 0 0 0 0 1 1 1 1
  line L28 (-25.1414, -8.2284) -> (-24.9274, -7.7201)
  line L29 (-24.9274, -7.7201) -> (-25.2733, -6.9429)
  spline S251 degree 3 poles (-25.2733, -6.9429) (-25.469, -6.5206) (-25.7161, -6.0436) (-25.8266, -5.8843) knots 0 0 0 0 1 1 1 1
  spline S252 degree 3 poles (-25.8266, -5.8843) (-26.1378, -5.462) (-26.7579, -3.6717) (-26.8998, -2.8203) knots 0 0 0 0 1 1 1 1
  spline S253 degree 3 poles (-26.8998, -2.8203) (-27.1143, -1.4809) (-27.2276, -0.3041) (-27.1839, 0.0374) knots 0 0 0 0 1 1 1 1
  spline S254 degree 3 poles (-27.1839, 0.0374) (-27.1578, 0.2254) (-27.1411, 0.641) (-27.1496, 0.9529) knots 0 0 0 0 1 1 1 1
  spline S255 degree 3 poles (-27.1496, 0.9529) (-27.1581, 1.2648) (-27.1136, 1.6905) (-27.0504, 1.892) knots 0 0 0 0 1 1 1 1
  spline S256 degree 3 poles (-27.0504, 1.892) (-26.9872, 2.0935) (-26.9309, 2.429) (-26.9301, 2.6288) knots 0 0 0 0 1 1 1 1
  spline S257 degree 3 poles (-26.9301, 2.6288) (-26.92, 2.832) (-26.8822, 3.1607) (-26.8283, 3.3589) knots 0 0 0 0 1 1 1 1
  spline S258 degree 3 poles (-26.8283, 3.3589) (-26.7837, 3.5536) (-26.7096, 3.9271) (-26.6574, 4.1876) knots 0 0 0 0 1 1 1 1
  spline S259 degree 3 poles (-26.6574, 4.1876) (-26.6086, 4.4573) (-26.4932, 4.9193) (-26.4014, 5.2153) knots 0 0 0 0 1 1 1 1
  spline S260 degree 3 poles (-26.4014, 5.2153) (-26.3037, 5.5238) (-26.1674, 6.13) (-26.0798, 6.5819) knots 0 0 0 0 1 1 1 1
  spline S261 degree 3 poles (-26.0798, 6.5819) (-25.9771, 7.1652) (-25.7404, 7.7554) (-25.2282, 8.7714) knots 0 0 0 0 1 1 1 1
  spline S262 degree 3 poles (-25.2282, 8.7714) (-24.5348, 10.1263) (-24.4346, 10.5722) (-24.8426, 10.4237) knots 0 0 0 0 1 1 1 1
  spline S263 degree 3 poles (-24.8426, 10.4237) (-24.9539, 10.3832) (-25.2968, 9.7964) (-25.7248, 8.8951) knots 0 0 0 0 1 1 1 1
  spline S264 degree 3 poles (-25.7248, 8.8951) (-26.3094, 7.6743) (-26.4502, 7.4551) (-26.5985, 7.5166) knots 0 0 0 0 1 1 1 1
  spline S265 degree 3 poles (-26.5985, 7.5166) (-26.6904, 7.5671) (-27.0817, 8.0652) (-27.4781, 8.635) knots 0 0 0 0 1 1 1 1
  spline S266 degree 3 poles (-27.4781, 8.635) (-27.8618, 9.1988) (-28.2304, 9.6632) (-28.302, 9.6581) knots 0 0 0 0 1 1 1 1
  spline S267 degree 3 poles (-28.302, 9.6581) (-28.5827, 9.6505) (-28.101, 8.3558) (-27.498, 7.5357) knots 0 0 0 0 1 1 1 1
  spline S268 degree 3 poles (-27.498, 7.5357) (-27.401, 7.4135) (-27.4592, 7.3713) (-27.9042, 7.2093) knots 0 0 0 0 1 1 1 1
  spline S269 degree 3 poles (-27.9042, 7.2093) (-28.1917, 7.1047) (-28.4302, 7.0389) (-28.437, 7.0574) knots 0 0 0 0 1 1 1 1
  spline S270 degree 3 poles (-28.437, 7.0574) (-28.4437, 7.076) (-28.4438, 7.307) (-28.4228, 7.5666) knots 0 0 0 0 1 1 1 1
  spline S271 degree 3 poles (-28.4228, 7.5666) (-28.3977, 8.1323) (-28.5798, 8.402) (-28.9811, 8.3504) knots 0 0 0 0 1 1 1 1
  spline S272 degree 3 poles (-28.9811, 8.3504) (-30.0542, 8.2119) (-30.0542, 8.2119) (-29.9236, 8.4589) knots 0 0 0 0 1 1 1 1
  spline S273 degree 3 poles (-29.9236, 8.4589) (-29.8553, 8.5888) (-29.7357, 8.7793) (-29.6447, 8.8754) knots 0 0 0 0 1 1 1 1
  spline S274 degree 3 poles (-29.6447, 8.8754) (-29.4812, 9.0609) (-29.3954, 9.6907) (-29.4966, 9.9688) knots 0 0 0 0 1 1 1 1
  spline S275 degree 3 poles (-29.4966, 9.9688) (-29.5236, 10.043) (-29.6518, 10.1644) (-29.769, 10.2267) knots 0 0 0 0 1 1 1 1
  spline S276 degree 3 poles (-29.769, 10.2267) (-29.9907, 10.3455) (-29.9848, 10.3582) (-29.8357, 10.6119) knots 0 0 0 0 1 1 1 1
  spline S277 degree 3 poles (-29.8357, 10.6119) (-29.4709, 11.1962) (-28.8852, 11.8084) (-28.6829, 11.8296) knots 0 0 0 0 1 1 1 1
  spline S278 degree 3 poles (-28.6829, 11.8296) (-28.4367, 11.8457) (-28.1932, 12.3018) (-28.0914, 12.9164) knots 0 0 0 0 1 1 1 1
  spline S279 degree 3 poles (-28.0914, 12.9164) (-27.8322, 14.5122) (-26.9939, 16.1614) (-25.9118, 17.2272) knots 0 0 0 0 1 1 1 1
  spline S280 degree 3 poles (-25.9118, 17.2272) (-25.2494, 17.8883) (-24.0147, 18.6213) (-23.1819, 18.8719) knots 0 0 0 0 1 1 1 1
  spline S281 degree 3 poles (-23.1819, 18.8719) (-21.389, 19.3984) (-20.4128, 19.4282) (-18.5884, 19.0317) knots 0 0 0 0 1 1 1 1
  line L30 (-18.5884, 19.0317) -> (-18.1079, 18.9231)
  line L31 (-18.1079, 18.9231) -> (-18.8083, 18.3952)
  spline S282 degree 3 poles (-18.8083, 18.3952) (-20.4871, 17.1226) (-21.2877, 16.2642) (-21.1561, 15.9026) knots 0 0 0 0 1 1 1 1
  spline S283 degree 3 poles (-21.1561, 15.9026) (-21.0549, 15.6245) (-20.7506, 15.7982) (-19.3221, 16.9797) knots 0 0 0 0 1 1 1 1
  spline S284 degree 3 poles (-19.3221, 16.9797) (-17.6921, 18.3289) (-17.0237, 18.7717) (-15.6128, 19.4533) knots 0 0 0 0 1 1 1 1
  spline S285 degree 3 poles (-15.6128, 19.4533) (-14.5592, 19.9627) (-12.2142, 20.8477) (-11.3308, 21.0748) knots 0 0 0 0 1 1 1 1
  spline S286 degree 3 poles (-11.3308, 21.0748) (-11.0147, 21.1583) (-10.1904, 21.3744) (-9.5118, 21.5583) knots 0 0 0 0 1 1 1 1
  spline S287 degree 3 poles (-9.5118, 21.5583) (-8.824, 21.7457) (-7.815, 21.9449) (-7.2645, 22.0193) knots 0 0 0 0 1 1 1 1
  spline S288 degree 3 poles (-7.2645, 22.0193) (-6.0945, 22.1511) (-3.4391, 22.1831) (-3.1296, 22.0542) knots 0 0 0 0 1 1 1 1
  spline S289 degree 3 poles (-3.1296, 22.0542) (-3.0192, 22.0104) (-2.875, 21.9894) (-2.8194, 22.0096) knots 0 0 0 0 1 1 1 1
  spline S290 degree 3 poles (-2.8194, 22.0096) (-2.7638, 22.0299) (-2.6415, 22.0114) (-2.5496, 21.9608) knots 0 0 0 0 1 1 1 1
  spline S291 degree 3 poles (-2.5496, 21.9608) (-2.4518, 21.9229) (-1.9907, 21.8387) (-1.5211, 21.7891) knots 0 0 0 0 1 1 1 1
  spline S292 degree 3 poles (-1.5211, 21.7891) (-0.8105, 21.7118) (-0.6671, 21.7219) (-0.6335, 21.8602) knots 0 0 0 0 1 1 1 1
  spline S293 degree 3 poles (-0.6335, 21.8602) (-0.5729, 22.1553) (-0.7356, 22.285) (-1.1959, 22.338) knots 0 0 0 0 1 1 1 1
  spline S294 degree 3 poles (-1.1959, 22.338) (-1.437, 22.3658) (-1.7852, 22.428) (-1.9833, 22.4819) knots 0 0 0 0 1 1 1 1
  spline S295 degree 3 poles (-1.9833, 22.4819) (-2.1688, 22.5299) (-2.479, 22.5745) (-2.6602, 22.5821) knots 0 0 0 0 1 1 1 1
  spline S296 degree 3 poles (-2.6602, 22.5821) (-2.8541, 22.5955) (-3.0236, 22.6283) (-3.0405, 22.6747) knots 0 0 0 0 1 1 1 1
  spline S297 degree 3 poles (-3.0405, 22.6747) (-3.054, 22.7118) (-2.8096, 23.0212) (-2.4969, 23.345) knots 0 0 0 0 1 1 1 1
  spline S298 degree 3 poles (-2.4969, 23.345) (-2.1843, 23.6688) (-1.9003, 24.0137) (-1.8716, 24.1081) knots 0 0 0 0 1 1 1 1
  spline S299 degree 3 poles (-1.8716, 24.1081) (-1.8396, 24.1933) (-1.7672, 24.2826) (-1.7208, 24.2995) knots 0 0 0 0 1 1 1 1
  spline S300 degree 3 poles (-1.7208, 24.2995) (-1.6652, 24.3198) (-1.511, 24.5019) (-1.3761, 24.7085) knots 0 0 0 0 1 1 1 1
  spline S301 degree 3 poles (-1.3761, 24.7085) (-1.2447, 24.9243) (-1.0121, 25.2085) (-0.8663, 25.356) knots 0 0 0 0 1 1 1 1
  spline S302 degree 3 poles (-0.8663, 25.356) (1.0391, 27.2466) (2.3698, 28.8124) (2.6452, 29.4692) knots 0 0 0 0 1 1 1 1
  spline S303 degree 3 poles (2.6452, 29.4692) (2.7033, 29.6269) (2.7521, 30.1276) (2.7461, 30.5769) knots 0 0 0 0 1 1 1 1
  spline S304 degree 3 poles (2.7461, 30.5769) (2.7434, 31.017) (2.7644, 31.3921) (2.8015, 31.4056) knots 0 0 0 0 1 1 1 1
  spline S305 degree 3 poles (2.8015, 31.4056) (2.8293, 31.4157) (3.0569, 31.3096) (3.3166, 31.1731) knots 0 0 0 0 1 1 1 1
  spline S306 degree 3 poles (3.3166, 31.1731) (3.6842, 30.9709) (3.8756, 30.9355) (4.2701, 31.0056) knots 0 0 0 0 1 1 1 1
  spline S307 degree 3 poles (4.2701, 31.0056) (4.6679, 31.0664) (4.8003, 31.1356) (4.9452, 31.3144) knots 0 0 0 0 1 1 1 1
  spline S308 degree 3 poles (4.9452, 31.3144) (5.1828, 31.6423) (5.6395, 32.6381) (5.7312, 33.0495) knots 0 0 0 0 1 1 1 1
  line L32 (5.7312, 33.0495) -> (5.8061, 33.3917)
  line L33 (5.8061, 33.3917) -> (6.1292, 32.8793)
  spline S309 degree 3 poles (6.1292, 32.8793) (6.2962, 32.5936) (6.5576, 32.0482) (6.7087, 31.6622) knots 0 0 0 0 1 1 1 1
  spline S310 degree 3 poles (6.7087, 31.6622) (6.9719, 30.939) (7.2097, 30.6895) (7.406, 30.929) knots 0 0 0 0 1 1 1 1
  spline S311 degree 3 poles (7.406, 30.929) (7.4482, 30.9863) (7.7415, 31.2191) (8.0727, 31.4341) knots 0 0 0 0 1 1 1 1
  line L34 (8.0727, 31.4341) -> (8.6517, 31.8339)
  line L35 (8.6517, 31.8339) -> (8.6577, 31.6156)
  spline S312 degree 3 poles (8.6577, 31.6156) (8.6611, 31.4908) (8.6215, 31.2244) (8.5643, 31.0355) knots 0 0 0 0 1 1 1 1
  spline S313 degree 3 poles (8.5643, 31.0355) (8.3984, 30.4816) (8.3025, 29.7642) (8.2109, 28.5444) knots 0 0 0 0 1 1 1 1
  spline S314 degree 3 poles (8.2109, 28.5444) (8.1211, 27.3777) (7.909, 26.1139) (7.5613, 24.6749) knots 0 0 0 0 1 1 1 1
  spline S315 degree 3 poles (7.5613, 24.6749) (7.4518, 24.2255) (7.3711, 23.7551) (7.3711, 23.6396) knots 0 0 0 0 1 1 1 1
  spline S316 degree 3 poles (7.3711, 23.6396) (7.3838, 23.5182) (7.2726, 23.0158) (7.1303, 22.5124) knots 0 0 0 0 1 1 1 1
  spline S317 degree 3 poles (7.1303, 22.5124) (6.9973, 22.0125) (6.8499, 21.3499) (6.8273, 21.0371) knots 0 0 0 0 1 1 1 1
  spline S318 degree 3 poles (6.8273, 21.0371) (6.7987, 20.7117) (6.7094, 20.4377) (6.6353, 20.4107) knots 0 0 0 0 1 1 1 1
  spline S319 degree 3 poles (6.6353, 20.4107) (6.5518, 20.3803) (6.2146, 20.3836) (5.8707, 20.4054) knots 0 0 0 0 1 1 1 1
  spline S320 degree 3 poles (5.8707, 20.4054) (5.5267, 20.4272) (5.1592, 20.3985) (5.0454, 20.3361) knots 0 0 0 0 1 1 1 1
  spline S321 degree 3 poles (5.0454, 20.3361) (4.7285, 20.1682) (4.839, 19.8934) (5.2959, 19.7342) knots 0 0 0 0 1 1 1 1
  spline S322 degree 3 poles (5.2959, 19.7342) (6.2916, 19.3931) (8.3564, 18.3071) (8.9821, 17.7998) knots 0 0 0 0 1 1 1 1
  spline S323 degree 3 poles (8.9821, 17.7998) (9.3522, 17.504) (9.8405, 17.1147) (10.0513, 16.9394) knots 0 0 0 0 1 1 1 1
  spline S324 degree 3 poles (10.0513, 16.9394) (10.5395, 16.5501) (10.8413, 16.471) (10.8909, 16.7095) knots 0 0 0 0 1 1 1 1
  spline S325 degree 3 poles (10.8909, 16.7095) (10.9238, 16.879) (10.7391, 17.2423) (10.5451, 17.3712) knots 0 0 0 0 1 1 1 1
  spline S326 degree 3 poles (10.5451, 17.3712) (10.4912, 17.404) (10.3529, 17.5532) (10.2491, 17.694) knots 0 0 0 0 1 1 1 1
  spline S327 degree 3 poles (10.2491, 17.694) (9.8907, 18.1305) (7.7803, 19.6304) (7.5088, 19.6261) knots 0 0 0 0 1 1 1 1
  spline S328 degree 3 poles (7.5088, 19.6261) (7.4153, 19.6236) (7.2264, 19.6809) (7.0932, 19.7584) knots 0 0 0 0 1 1 1 1
  line L36 (7.0932, 19.7584) -> (6.8462, 19.889)
  line L37 (6.8462, 19.889) -> (7.2963, 19.9793)
  spline S329 degree 3 poles (7.2963, 19.9793) (7.8147, 20.084) (9.8815, 20.9832) (12.3612, 22.1903) knots 0 0 0 0 1 1 1 1
  spline S330 degree 3 poles (12.3612, 22.1903) (15.7715, 23.841) (17.3232, 24.5108) (22.1732, 26.4756) knots 0 0 0 0 1 1 1 1
  spline S331 degree 3 poles (22.1732, 26.4756) (23.4823, 27.0045) (24.1911, 27.336) (24.2324, 27.4246) knots 0 0 0 0 1 1 1 1
  spline S332 degree 3 poles (24.2324, 27.4246) (24.2737, 27.5131) (24.3773, 27.6033) (24.4701, 27.6371) knots 0 0 0 0 1 1 1 1
  spline S333 degree 3 poles (24.4701, 27.6371) (24.6277, 27.6944) (24.6403, 27.6885) (24.5763, 27.4027) knots 0 0 0 0 1 1 1 1
  spline S334 degree 3 poles (24.5763, 27.4027) (24.5166, 27.192) (24.4744, 27.1346) (24.385, 27.2071) knots 0 0 0 0 1 1 1 1
  spline S335 degree 3 poles (-27.7102, -1.8342) (-27.6223, -2.7683) (-27.3378, -4.0403) (-27.0476, -4.8376) knots 0 0 0 0 1 1 1 1
  spline S336 degree 3 poles (-27.0476, -4.8376) (-26.9295, -5.1622) (-26.8535, -5.4285) (-26.8813, -5.4386) knots 0 0 0 0 1 1 1 1
  spline S337 degree 3 poles (-26.8813, -5.4386) (-26.9092, -5.4488) (-27.125, -5.4328) (-27.3568, -5.4017) knots 0 0 0 0 1 1 1 1
  spline S338 degree 3 poles (-27.3568, -5.4017) (-27.5853, -5.3798) (-28.0759, -5.3589) (-28.4409, -5.3658) knots 0 0 0 0 1 1 1 1
  spline S339 degree 3 poles (-28.4409, -5.3658) (-28.8059, -5.3726) (-29.1532, -5.3415) (-29.2072, -5.3087) knots 0 0 0 0 1 1 1 1
  spline S340 degree 3 poles (-29.2072, -5.3087) (-29.488, -5.0854) (-29.0097, -3.1682) (-28.3778, -1.9617) knots 0 0 0 0 1 1 1 1
  spline S341 degree 3 poles (-28.3778, -1.9617) (-28.1284, -1.493) (-27.9153, -1.0689) (-27.8824, -1.0149) knots 0 0 0 0 1 1 1 1
  spline S342 degree 3 poles (-27.8824, -1.0149) (-27.8176, -0.8758) (-27.799, -0.9845) (-27.7102, -1.8342) knots 0 0 0 0 1 1 1 1
  spline S343 degree 3 poles (5.898, 13.5797) (5.7167, 13.7027) (5.6889, 13.6926) (5.1807, 13.3291) knots 0 0 0 0 1 1 1 1
  line L38 (5.1807, 13.3291) -> (4.6446, 12.9555)
  line L39 (4.6446, 12.9555) -> (4.3782, 13.1106)
  spline S344 degree 3 poles (4.3782, 13.1106) (3.8167, 13.4417) (3.6742, 13.5158) (3.299, 13.6523) knots 0 0 0 0 1 1 1 1
  spline S345 degree 3 poles (3.299, 13.6523) (2.6085, 13.905) (1.3903, 14.1651) (0.7184, 14.1936) knots 0 0 0 0 1 1 1 1
  spline S346 degree 3 poles (0.7184, 14.1936) (-0.085, 14.2372) (-1.4379, 13.9442) (-2.3693, 13.5317) knots 0 0 0 0 1 1 1 1
  spline S347 degree 3 poles (-2.3693, 13.5317) (-3.2636, 13.1327) (-3.7953, 12.6032) (-4.2587, 11.626) knots 0 0 0 0 1 1 1 1
  spline S348 degree 3 poles (-4.2587, 11.626) (-5.0355, 10.0098) (-5.0671, 8.6542) (-4.3718, 6.5132) knots 0 0 0 0 1 1 1 1
  spline S349 degree 3 poles (-4.3718, 6.5132) (-4.0031, 5.3559) (-3.9432, 5.2202) (-3.7839, 5.2152) knots 0 0 0 0 1 1 1 1
  spline S350 degree 3 poles (-3.7839, 5.2152) (-3.5091, 5.2102) (-2.2879, 6.2112) (-1.1822, 7.3277) knots 0 0 0 0 1 1 1 1
  spline S351 degree 3 poles (-1.1822, 7.3277) (-0.7937, 7.7316) (0.0306, 8.4096) (0.6526, 8.8355) knots 0 0 0 0 1 1 1 1
  spline S352 degree 3 poles (0.6526, 8.8355) (1.2619, 9.2673) (2.1207, 9.9369) (2.5598, 10.3172) knots 0 0 0 0 1 1 1 1
  spline S353 degree 3 poles (2.5598, 10.3172) (2.9989, 10.6975) (3.5273, 11.1208) (3.7263, 11.2667) knots 0 0 0 0 1 1 1 1
  spline S354 degree 3 poles (3.7263, 11.2667) (3.9285, 11.4034) (4.1451, 11.5872) (4.2151, 11.6547) knots 0 0 0 0 1 1 1 1
  spline S355 degree 3 poles (4.2151, 11.6547) (4.2816, 11.7314) (4.6845, 12.067) (5.1185, 12.4035) knots 0 0 0 0 1 1 1 1
  spline S356 degree 3 poles (5.1185, 12.4035) (6.0203, 13.0992) (6.2032, 13.3758) (5.898, 13.5797) knots 0 0 0 0 1 1 1 1
  spline S357 degree 3 poles (2.6, 11.3608) (0.2048, 9.46) (-0.1113, 9.261) (-0.8717, 9.2152) knots 0 0 0 0 1 1 1 1
  spline S358 degree 3 poles (-0.8717, 9.2152) (-1.6852, 9.1711) (-2.2861, 8.7739) (-2.1444, 8.3845) knots 0 0 0 0 1 1 1 1
  spline S359 degree 3 poles (-2.1444, 8.3845) (-2.0701, 8.1805) (-1.9099, 8.1443) (-1.4564, 8.2254) knots 0 0 0 0 1 1 1 1
  spline S360 degree 3 poles (-1.4564, 8.2254) (-1.0771, 8.2794) (-1.0712, 8.2921) (-1.9241, 7.6351) knots 0 0 0 0 1 1 1 1
  spline S361 degree 3 poles (-1.9241, 7.6351) (-2.2326, 7.3864) (-2.6472, 7.0254) (-2.8352, 6.8205) knots 0 0 0 0 1 1 1 1
  spline S362 degree 3 poles (-2.8352, 6.8205) (-3.2228, 6.3854) (-3.4571, 6.2791) (-3.6148, 6.4528) knots 0 0 0 0 1 1 1 1
  spline S363 degree 3 poles (-3.6148, 6.4528) (-3.673, 6.5261) (-3.835, 7.0866) (-3.9642, 7.7011) knots 0 0 0 0 1 1 1 1
  spline S364 degree 3 poles (-3.9642, 7.7011) (-4.2014, 8.8433) (-4.1866, 10.0142) (-3.938, 10.3987) knots 0 0 0 0 1 1 1 1
  spline S365 degree 3 poles (-3.938, 10.3987) (-3.8782, 10.494) (-3.7434, 10.8161) (-3.633, 11.1187) knots 0 0 0 0 1 1 1 1
  spline S366 degree 3 poles (-3.633, 11.1187) (-3.4048, 11.7898) (-2.6598, 12.628) (-2.0159, 12.9359) knots 0 0 0 0 1 1 1 1
  spline S367 degree 3 poles (-2.0159, 12.9359) (-1.1654, 13.3399) (1.2202, 13.5362) (2.0675, 13.2566) knots 0 0 0 0 1 1 1 1
  spline S368 degree 3 poles (2.0675, 13.2566) (2.9552, 12.9812) (3.7773, 12.5978) (3.8026, 12.4706) knots 0 0 0 0 1 1 1 1
  spline S369 degree 3 poles (3.8026, 12.4706) (3.8111, 12.3896) (3.2902, 11.9166) (2.6, 11.3608) knots 0 0 0 0 1 1 1 1
  spline S370 degree 3 poles (8.0704, -9.2657) (7.954, -9.2345) (7.4844, -8.8384) (6.201, -7.678) knots 0 0 0 0 1 1 1 1
  spline S371 degree 3 poles (6.201, -7.678) (5.7659, -7.2904) (5.2928, -6.885) (5.1529, -6.789) knots 0 0 0 0 1 1 1 1
  spline S372 degree 3 poles (5.1529, -6.789) (5.0095, -6.6836) (4.8755, -6.5749) (4.8653, -6.5471) knots 0 0 0 0 1 1 1 1
  spline S373 degree 3 poles (4.8653, -6.5471) (4.8417, -6.4822) (3.9926, -5.7937) (2.985, -5.0159) knots 0 0 0 0 1 1 1 1
  spline S374 degree 3 poles (2.985, -5.0159) (2.6342, -4.7446) (2.146, -4.3553) (1.9158, -4.1555) knots 0 0 0 0 1 1 1 1